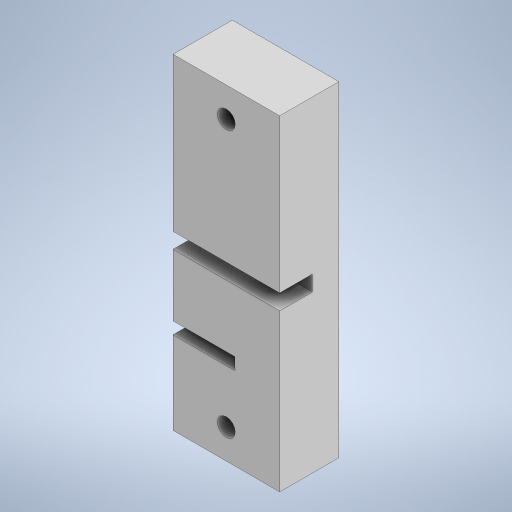
# Autodesk Inventor part: ジョイントモーターハメ
Saved by Autodesk Inventor 2023 (Build 270158000, 158)
## iProperties
Created: 2023-10-22
Part Number: ジョイントモーターハメ
Material: 一般
Document SubType Name: Modeling
Designer: ukkun
Density: 1 g/cm^3
Appearance: 既定
Author: ukkun
Autodesk Inventor part; units mm, degrees
ref_plane "YZ Plane" through (0, 0, 0) normal (1, 0, 0) x (0, 1, 0)
ref_plane "XZ Plane" through (0, 0, 0) normal (0, 1, 0) x (-1, 0, 0)
ref_plane "XY Plane" through (0, 0, 0) normal (0, 0, 1) x (1, 0, 0)
sketch "スケッチ1" plane through (0, 0, 0) normal (0, 0, 1) x (1, 0, 0)
  line L0 (-9, -27.5) -> (9, -27.5)
  line L1 (9, -27.5) -> (9, 27.5)
  line L2 (9, 27.5) -> (-9, 27.5)
  line L3 (-9, 27.5) -> (-9, -27.5)
  line L4 (-9, -27.5) -> (9, 27.5) construction
  line L5 (9, -27.5) -> (-9, 27.5) construction
  point P0 (0, 0)
  dimension "d0" = 18
  dimension "d1" = 55
  constraints: 12 end point, 2 midpoint, 2 parallel, 1 horizontal, 1 perpendicular
  measures "d0" distance of L1.end L2.end
  measures "d1" distance of L0.end L1.end
extrude "押し出し1" add sketch "スケッチ1" along normal blind 10
sketch "スケッチ2" plane through (0, 0, 10) normal (0, 0, 1) x (1, 0, 0)
  line L0 (-9, 27.5) -> (-9, -27.5) projected
  line L1 (9, -27.5) -> (9, 27.5) projected
  line L2 (-9, -1) -> (9, -1)
  line L3 (9, -1) -> (9, 1.6)
  line L4 (9, 1.6) -> (-9, 1.6)
  line L5 (-9, 1.6) -> (-9, -1)
  line L6 (-9, -27.5) -> (9, -27.5) projected
  point P0 (0, 0)
  point P1 (9, -1)
  dimension "d4" = 2.6
  dimension "d5" = 26.5
  constraints: 8 end point, 2 parallel, 2 point on line, 1 horizontal, 1 perpendicular
  measures "d4" distance between parallel lines of L2 L4
  measures "d5" distance between parallel lines of L6 L2
extrude "押し出し2" cut sketch "スケッチ2" against normal blind 5.5 contours L4 L1 L2 L0
sketch "スケッチ3" plane through (0, 0, 10) normal (0, 0, 1) x (1, 0, 0)
  line L0 (-9, -1) -> (-9, -27.5) projected
  line L1 (-9, -13.5) -> (1.45, -13.5)
  line L2 (1.45, -13.5) -> (1.45, -11.5)
  line L3 (1.45, -11.5) -> (-9, -11.5)
  line L4 (-9, -11.5) -> (-9, -13.5)
  line L5 (-9, -27.5) -> (9, -27.5) projected
  point P0 (0, 0)
  dimension "d8" = 2
  dimension "d9" = 14
  dimension "d10" = 10.45
  constraints: 8 end point, 2 parallel, 1 horizontal, 1 perpendicular, 1 point on line
  measures "d8" distance between parallel lines of L1 L3
  measures "d9" distance between parallel lines of L5 L1
  measures "d10" distance of L1.start L1.end
extrude "押し出し3" cut sketch "スケッチ3" against normal through all
sketch "スケッチ4" plane through (0, 0, 10) normal (0, 0, 1) x (1, 0, 0)
  circle A0 centre (0, 22.5) radius 1.5
  circle A1 centre (0, -22.5) radius 1.5
  line L0 (9, 27.5) -> (-9, 27.5) projected
  line L1 (-9, -27.5) -> (9, -27.5) projected
  point P0 (0, 0)
  dimension "d13" = 3
  dimension "d14" = 3
  dimension "d15" = 5
  dimension "d16" = 5
  constraints: 2 centre point
  measures "d13" diameter of A0
  measures "d14" diameter of A1
  measures "d15" distance from line of L0 A0.centre
  measures "d16" distance from line of L1 A1.centre
extrude "押し出し4" cut sketch "スケッチ4" against normal through all
